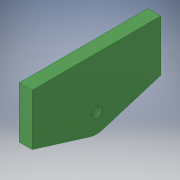
# Autodesk Inventor part: pivot plate
Saved by Autodesk Inventor 2017 SP1 (Build 210196100, 196)
## iProperties
Created: 2018-01-27
Part Number: pivot plate
Material: Generic
Document SubType Name: Modeling
Designer: Ben
Density: 1 g/cm^3
Appearance: Smooth - Dark Forest Green
Author: Ben
Autodesk Inventor part; units mm, degrees
ref_plane "YZ Plane" through (0, 0, 0) normal (1, 0, 0) x (0, 1, 0)
ref_plane "XZ Plane" through (0, 0, 0) normal (0, 1, 0) x (-1, 0, 0)
ref_plane "XY Plane" through (0, 0, 0) normal (0, 0, 1) x (1, 0, 0)
sketch "Sketch1" plane through (0, 0, 0) normal (1, 0, 0) x (0, 1, 0)
  circle A0 centre (0, 0) radius 2.54
  arc A1 (-9.1021, 2.8065) -> (-9.1021, -2.8065) centre (0, 0) ccw
  line L0 (-9.1021, 2.8065) -> (-0.1778, 31.75)
  line L1 (-0.1778, 31.75) -> (25.2222, 31.75)
  line L2 (25.2222, 31.75) -> (25.2222, -31.75)
  line L3 (25.2222, -31.75) -> (-0.1778, -31.75)
  line L4 (-0.1778, -31.75) -> (-9.1021, -2.8065)
  line L5 (12.5222, -31.75) -> (12.5222, 31.75) construction
  dimension "d0" = 5.08
  dimension "d1" = 25.4
  dimension "d2" = 12.5222
  dimension "d3" = 9.525
  dimension "d4" = 63.5
  constraints: 12 end point, 2 centre point, 2 coincident, 2 equal length, 2 midpoint, 2 point on circle, 2 tangent, 1 horizontal, 1 perpendicular, 1 vertical
  measures "d0" diameter of A0
  measures "d1" distance of L2.end L3.end
  measures "d2" distance from line of point (0, 0) L5
  measures "d3" radius of A1
  measures "d4" distance of L1.end L2.end
extrude "Extrusion1" add sketch "Sketch1" along normal blind 6.35
body "Solid1"
